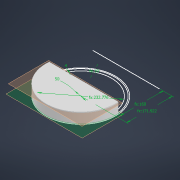
# Autodesk Inventor part: ballInletCover
Saved by Autodesk Inventor 2021.4 (Build 254397000, 397)
## iProperties
Created: 2022-04-06
Part Number: ballInletCover
Material: Generic
Document SubType Name: Modeling
Designer: jo_ki
Density: 1 g/cm^3
Appearance: Default
Author: jo_ki
Autodesk Inventor part; units mm, degrees
ref_plane "YZ Plane" through (0, 0, 0) normal (1, 0, 0) x (0, 1, 0)
ref_plane "XZ Plane" through (0, 0, 0) normal (0, 1, 0) x (-1, 0, 0)
ref_plane "XY Plane" through (0, 0, 0) normal (0, 0, 1) x (1, 0, 0)
sketch "Sketch1" plane through (0, 0, 0) normal (0, 1, 0) x (-1, 0, 0)
  circle A0 centre (0, 0) radius 116.3878
  circle A1 centre (0, 0) radius 126.3878
  line L0 (129.8416, -11.9217) -> (-129.8416, -11.9217)
  line L1 (125.8243, -171.9217) -> (-125.8243, -171.9217)
  circle A2 centre (0, 0) radius 130.3878
  circle A3 centre (0, 0) radius 25
  point P0 (-115.7756, -11.9217)
  point P1 (115.7756, -11.9217)
  point P2 (-125.8243, -11.9217)
  point P3 (125.8243, -11.9217)
  point P4 (-21.9744, -11.9217)
  point P5 (21.9744, -11.9217)
  dimension "d1" = 232.7756
  dimension "d2" = 10
  dimension "d6" = 160
  dimension "d7" = 171.9217
  dimension "d11" = 4
  dimension "d13" = 50
  constraints: 4 centre point, 4 coincident, 4 end point, 2 horizontal, 2 point on circle
  measures "d1" diameter of A0
  measures "d2" radial gap between concentric circles of A1 A0
  measures "d6" distance between parallel lines of L0 L1
  measures "d7" distance from line of point (0, 0) L1
  measures "d11" radial gap between concentric circles of A1 A2
  measures "d13" diameter of A3
extrude "Extrusion1" add sketch "Sketch1" along normal blind 40 contours A0 L0 A3 | A0 L0 A1 | A3 L0 | L0 A2 A1 picked at (-80.805, 28.5699) picked at (-122.0572, 13.8082) picked at (7.5455, -2.0688) picked at (1.8738, 127.5443)
ref_plane "Work Plane2" through (0, 37, 0) normal (0, 1, 0) x (1, 0, 0)
ref_plane "Work Plane3" through (0, 3, 0) normal (0, -1, 0) x (1, 0, 0)
extrude "Extrusion2" cut sketch "Sketch1" along normal up to surface (34 mm away) from surface at 3 contours A0 L0 A3 | A0 L0 A1 | A3 L0 picked at (-80.805, 28.5699) picked at (-122.0572, 13.8082) picked at (7.5455, -2.0688)
extrude "Extrusion3" cut sketch "Sketch1" along normal up to surface (3 mm away) contours A3 L0 picked at (7.5455, -2.0688)
equation "\"d1\" = ballInletWheel_diameter"
equation "\"d2\" = ballInletWheel_margin"
equation "\"d6\" = profile_height"
equation "\"d7\" = ballInletWheel_offsetTop"
equation "\"d3\" = profile_width"
equation "\"d14\" = profile_width"
equation "\"d8\" = -profileTallWall_thickness"
equation "\"d12\" = -profileTallWall_thickness"
equation "\"ballInletWheel_diameter\" = 232.775591"
equation "\"ballInletWheel_margin\" = 10"
equation "\"profile_height\" = 160"
equation "\"profile_width\" = 40"
equation "\"profileTallWall_thickness\" = 3"
equation "\"ballInletWheel_offsetTop\" = 171.921659"
body "Solid2"
